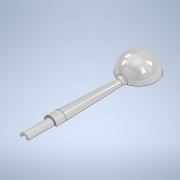
# Autodesk Inventor part: markerWithRodEnd
Saved by Autodesk Inventor 2022 (Build 260153000, 153)
## iProperties
Created: 2021-09-13
Part Number: markerWithRodEnd
Material: ABS Plastic
Document SubType Name: Modeling
Designer: tecware
Density: 1.06 g/cm^3
Appearance: Aluminum - Polished
Author: tecware
## iProperties of the stored document markerWithRodEnd_3DPrint.ipt
Created: 2021-09-13
Part Number: markerWithRodEnd_3DPrint
Material: Generic
Document SubType Name: Modeling
Designer: tecware
Density: 1 g/cm^3
Appearance: Default
Author: tecware
Autodesk Inventor part; units mm, degrees
ref_plane "YZ Plane" through (0, 0, 0) normal (1, 0, 0) x (0, 1, 0)
ref_plane "XZ Plane" through (0, 0, 0) normal (0, 1, 0) x (-1, 0, 0)
ref_plane "XY Plane" through (0, 0, 0) normal (0, 0, 1) x (1, 0, 0)
sketch "Sketch1" plane through (0, 0, 0) normal (0, 1, 0) x (-1, 0, 0)
  line L0 (0, 0) -> (-1.5, 0)
  line L1 (-1.5, 0) -> (-3.5, 0)
  line L2 (0, 0) -> (0, -40.75)
  line L3 (0, -40.75) -> (0, -50.75)
  circle A0 centre (0, -50.75) radius 10
  line L4 (-1.5, -40.8631) -> (0, -40.8631)
  line L5 (0, -40.8631) -> (0, -40.75)
  line L6 (-1.5, -40.8631) -> (-1.5, 0)
  line L7 (0, -40.75) -> (-1.5, -40.75)
  line L8 (-1.5, -40.75) -> (-2, -40.75)
  line L9 (0, -50.75) -> (0, -60.75)
  circle A1 centre (0, -50.75) radius 9.2
  line L10 (-1.5, 0) -> (-1.5, 15)
  line L11 (-3.5, 0) -> (-3.5, 15)
  line L12 (-3.5, 15) -> (-1.5, 15)
  arc A2 (-3.3801, -41.3386) -> (-2.0575, -39.3831) centre (-4.0561, -39.4563) ccw
  line L13 (-1.5, -40.8631) -> (-1.5, -41.6731)
  line L14 (0, 0) -> (-2.4, 0)
  line L15 (-2.4, 0) -> (-2.4, 15)
  line L16 (0, 0) -> (-1.5, 0)
  line L17 (-1.5, 0) -> (-1.5, 15)
  line L18 (-2.4, 15) -> (0, 15)
  line L19 (0, 15) -> (0, 0)
  line L20 (-1.5, 0) -> (-1.5, 0)
  line L21 (-1.5, 0) -> (-1.5, -2)
  line L22 (-1.5, -2) -> (-1.5, -2)
  line L23 (-3.5, 0) -> (-3.5, -5.75)
  line L24 (-3.5, -5.75) -> (-2.0575, -39.3831)
  point P0 (0, -59.95)
  point P1 (0, -41.55)
  dimension "d7" = 18.4
  dimension "d1" = 2
  dimension "d2" = 40.75
  dimension "d4" = 10
  dimension "d9" = 15
  dimension "d16" = 1.5
  dimension "d19" = 2
  dimension "d20" = 2.4
  dimension "d21" = 15
  dimension "d22" = 1.5
  dimension "d23" = 2
  dimension "d24" = 3.5
  dimension "d25" = 5.75
  constraints: 50 end point, 7 point on line, 6 point on circle, 4 vertical, 2 centre point, 2 coincident, 2 horizontal, 2 perpendicular, 2 tangent, 3 other
  measures "d1" distance of L0.end L1.end
  measures "d2" distance of L0.start L2.end
  measures "d4" distance of L2.end L3.end
  measures "d9" distance of L0.end L10.end
  measures "d16" distance of L4.start L4.end
  measures "d19" radius of A2
  measures "d20" distance of L0.start L14.end
  measures "d21" distance of L14.end L15.end
  measures "d22" distance of L0.start L16.end
  measures "d23" distance of L16.end L21.end
  measures "d24" distance between parallel lines of L19 L11
  measures "d25" distance of L1.end L23.end
revolve "Revolution1" add sketch "Sketch1" angle 180 about axis through (0, 0, 0) along (0, 0, 1) contours L6 A0 A2 L24 L23 L1 | L1 L15 L12 L10 | L13 A1 L9 A0
sketch "Sketch2" plane through (3.7, 0, 0) normal (0, 0, 1) x (1, 0, 0)
  circle A0 centre (-3.7, 0) radius 3.7
  circle A1 centre (-3.7, 0) radius 2.2
  line L0 (-0.2, 0) -> (-1.6425, 0) projected
  line L1 (0, 0) -> (-7.4, 0)
  point P0 (-1.7, 0)
  point P1 (-5.9, 0)
  point P2 (-1.5, 0)
  dimension "d13" = 4.4
  dimension "d14" = 7.4
  constraints: 2 centre point, 2 coincident, 2 end point, 2 point on circle, 1 collinear, 1 point on line
  measures "d13" diameter of A1
  measures "d14" diameter of A0
extrude "Rod Stopper" [suppressed]
equation "\"d23\" = d1"
body "Solid1"
